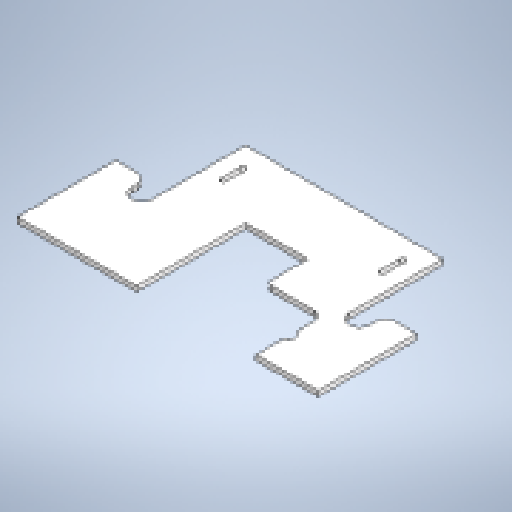
# Autodesk Inventor part: Top Plate
Saved by Autodesk Inventor 2023.4 (Build 274418000, 418)
## iProperties
Created: 2023-11-13
Part Number: Top Plate
Material: UHMW, White
Document SubType Name: Modeling
Designer: Nathan Cai
Density: 0.94 g/cm^3
Appearance: Smooth - White
Mass: 36.5863 g
Surface Area: 271.6 cm^2
Volume: 38.9216 cm^3
Author: Nathan Cai
Autodesk Inventor part; units mm, degrees
ref_plane "YZ Plane" through (0, 0, 0) normal (1, 0, 0) x (0, 1, 0)
ref_plane "XZ Plane" through (0, 0, 0) normal (0, 1, 0) x (-1, 0, 0)
ref_plane "XY Plane" through (0, 0, 0) normal (0, 0, 1) x (1, 0, 0)
sketch "Sketch1" plane through (0, 0, 0) normal (0, 1, 0) x (-1, 0, 0)
  line L0 (-60.325, 53.975) -> (60.325, 53.975)
  line L1 (60.325, 53.975) -> (60.325, -53.975)
  line L2 (60.325, -53.975) -> (-60.325, -53.975)
  line L3 (-60.325, -53.975) -> (-60.325, 53.975)
  line L4 (-60.325, 53.975) -> (60.325, -53.975) construction
  line L5 (60.325, 53.975) -> (-60.325, -53.975) construction
  line L6 (19.05, 120.65) -> (-19.05, 120.65)
  line L7 (-19.05, 120.65) -> (-19.05, -12.7)
  line L8 (-19.05, -12.7) -> (19.05, -12.7)
  line L9 (19.05, -12.7) -> (19.05, 120.65)
  line L10 (19.05, 120.65) -> (-19.05, -12.7) construction
  line L11 (-19.05, 120.65) -> (19.05, -12.7) construction
  line L12 (-19.05, 53.975) -> (-53.975, 53.975)
  line L13 (-53.975, 53.975) -> (-53.975, 12.7)
  line L14 (-53.975, 12.7) -> (-19.05, 12.7)
  line L15 (-19.05, 12.7) -> (-19.05, 53.975)
  line L16 (-48.7375, -28.575) -> (-48.7375, -41.275) construction
  line L17 (-50.325, -28.575) -> (-50.325, -41.275)
  line L18 (-47.15, -41.275) -> (-47.15, -28.575)
  arc A0 (-47.15, -28.575) -> (-50.325, -28.575) centre (-48.7375, -28.575) ccw
  arc A1 (-50.325, -41.275) -> (-47.15, -41.275) centre (-48.7375, -41.275) ccw
  line L19 (0, 0) -> (0, -53.975) construction
  line L20 (48.7375, -28.575) -> (48.7375, -41.275) construction
  line L21 (50.325, -28.575) -> (50.325, -41.275)
  line L22 (47.15, -41.275) -> (47.15, -28.575)
  arc A2 (50.325, -28.575) -> (47.15, -28.575) centre (48.7375, -28.575) ccw
  arc A3 (47.15, -41.275) -> (50.325, -41.275) centre (48.7375, -41.275) ccw
  line L23 (92.075, 53.975) -> (-92.075, 53.975)
  line L24 (-92.075, 53.975) -> (-92.075, -6.35)
  line L25 (-92.075, -6.35) -> (92.075, -6.35)
  line L26 (92.075, -6.35) -> (92.075, 53.975)
  line L27 (92.075, 53.975) -> (-92.075, -6.35) construction
  line L28 (-92.075, 53.975) -> (92.075, -6.35) construction
  line L29 (66.675, -15.875) -> (66.675, 3.175) construction
  line L30 (73.025, -15.875) -> (73.025, 3.175)
  line L31 (60.325, 3.175) -> (60.325, -15.875)
  arc A4 (60.325, -15.875) -> (73.025, -15.875) centre (66.675, -15.875) ccw
  arc A5 (73.025, 3.175) -> (60.325, 3.175) centre (66.675, 3.175) ccw
  line L32 (-66.675, -15.875) -> (-66.675, 3.175) construction
  line L33 (-73.025, -15.875) -> (-73.025, 3.175)
  line L34 (-60.325, 3.175) -> (-60.325, -15.875)
  arc A6 (-73.025, -15.875) -> (-60.325, -15.875) centre (-66.675, -15.875) ccw
  arc A7 (-60.325, 3.175) -> (-73.025, 3.175) centre (-66.675, 3.175) ccw
  circle A8 centre (-53.975, 33.3375) radius 3.175
  point P0 (0, 53.975)
  point P1 (19.05, 53.975)
  point P2 (-19.05, 53.975)
  point P3 (-19.05, 12.7)
  point P4 (-19.05, 53.975)
  point P5 (-53.975, 53.975)
  point P6 (-48.7375, -34.925)
  point P7 (48.7375, -34.925)
  point P8 (0, 23.8125)
  point P9 (66.675, -6.35)
  point P10 (-66.675, -6.35)
  point P11 (-73.025, -6.35)
  point P12 (-60.325, 3.175)
  point P13 (-60.325, 53.975)
  point P14 (60.325, 3.175)
  point P15 (73.025, -6.35)
  point P16 (-53.975, 30.1625)
  point P17 (-53.975, 36.5125)
  dimension "d0" = 120.65
  dimension "d1" = 107.95
  dimension "d4" = 38.1
  dimension "d5" = 133.35
  dimension "d11" = 34.925
  dimension "d12" = 41.275
  dimension "d13" = 0
  dimension "d16" = 3.175
  dimension "d17" = 10
  dimension "d18" = 12.7
  dimension "d19" = 19.05
  dimension "d20" = 184.15
  dimension "d21" = 60.325
  dimension "d22" = 19.05
  dimension "d23" = 9.525
  dimension "d25" = 6.35
  constraints: 78 end point, 16 point on circle, 14 symmetric about line, 12 midpoint, 10 parallel, 9 centre point, 9 tangent, 5 perpendicular, 4 horizontal, 3 point on line, 1 vertical, 4 other
  measures "d0" distance of L1.end L2.end
  measures "d1" distance of L0.end L1.end
  measures "d4" distance of L8.end L7.end
  measures "d5" distance of L7.end L6.end
  measures "d11" distance of L14.end L13.end
  measures "d12" distance of L13.end L12.end
  measures "d13" distance between parallel lines of L0 L12
  measures "d16" diameter of A1
  measures "d17" distance between parallel lines of L3 L17
  measures "d18" distance of L16.end L16.start
  measures "d19" distance from line of L2 point (-48.737, -34.925)
  measures "d20" distance of L25.end L24.end
  measures "d21" distance between parallel lines of L23 L25
  measures "d22" distance between parallel lines of L26 L30
  measures "d23" distance from line of L29.end L25
  measures "d25" diameter of A8
extrude "Extrusion1" add sketch "Sketch1" along normal blind 3.175 contours L0 L13 A8 L14 L7 L25 L3 | L3 A7 L33 L25 L24 L23 | L25 L7 L8 L9 L1 L2 L3 | L0 L1 L25 L9 | L23 L26 L25 L30 A5 L1
fillet "Fillet4" radius 3.175 1 edges at (19.05, 1.5875, 12.7)
fillet "Fillet5" radius 6.35 1 edges at (53.975, 1.5875, 12.7)
fillet "Fillet6" radius 6.35 2 edges at (73.025, 1.5875, -6.35) (-73.025, 1.5875, -6.35)
fillet "Fillet7" radius 3.175 2 edges at (53.975, 1.5875, 30.1625) (53.975, 1.5875, 36.5125)
body "Solid1"
